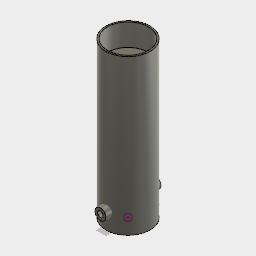
brazo (Autodesk Fusion 360 design; units mm, degrees)
Autodesk Fusion 360 part; units mm, degrees
sketch "Sketch1" plane through (0, 0, 0) normal (0, 1, 0) x (1, 0, 0)
  circle A0 centre (0, 0) radius 10
  dimension "d1" = 20
  measures "d1" diameter of A0
sketch "Sketch2" plane through (0, 0, 0) normal (0, 1, 0) x (1, 0, 0)
sketch "Sketch3" plane through (0, 0, 0) normal (0, 0, 1) x (1, 0, 0)
  circle A0 centre (0, 15) radius 5
  dimension "d10" = 10
  measures "d10" diameter of A0
sketch "Sketch4" plane through (0, 0, 0) normal (0, 1, 0) x (1, 0, 0)
  circle A0 centre (0, 0) radius 20
  dimension "d20" = 40
  measures "d20" diameter of A0
extrude "Extrude4" add sketch "Sketch4" along normal blind 140 makes body 1
sketch "Sketch5" plane through (0, 140, 0) normal (0, 1, 0) x (-1, 0, 0)
  circle A0 centre (0, 0) radius 20
  circle A1 centre (0, 0) radius 18.5
  dimension "d23" = 37
  measures "d23" diameter of A1
extrude "Extrude5" cut sketch "Sketch5" against normal blind 20 contours A1 bodies 1
sketch "Sketch6" plane through (0, 0, 0) normal (0, 0, 1) x (1, 0, 0)
  circle A0 centre (0, 15) radius 5
  dimension "d26" = 10
  measures "d26" diameter of A0
extrude "Extrude6" add sketch "Sketch6" along normal blind 25 and the other way blind 25 separate body makes body 2
sketch "Sketch7" plane through (0, 0, 25) normal (0, 0, 1) x (1, 0, 0)
  circle A0 centre (0, 15) radius 5
hole "Hole3" at (0, 15, 25) direction (0, 0, -1) diameter 5 depth 50 tip angle 118 bodies 1 2
